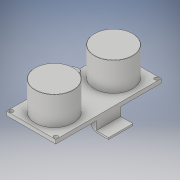
# Autodesk Inventor part: ultrasonicSensor
Saved by Autodesk Inventor 2018 (Build 220112000, 112)
## iProperties
Created: 2020-03-26
Part Number: ultrasonicSensor
Material: Generic
Document SubType Name: Modeling
Designer: natha
Density: 1 g/cm^3
Appearance: Default
Author: natha
Autodesk Inventor part; units mm, degrees
ref_plane "YZ Plane" through (0, 0, 0) normal (1, 0, 0) x (0, 1, 0)
ref_plane "XZ Plane" through (0, 0, 0) normal (0, 1, 0) x (-1, 0, 0)
ref_plane "XY Plane" through (0, 0, 0) normal (0, 0, 1) x (1, 0, 0)
sketch "Sketch1" plane through (0, 0, 0) normal (0, 1, 0) x (-1, 0, 0)
  line L0 (0, 0) -> (20.25, 0)
  line L1 (20.25, 0) -> (20.25, -43.35)
  line L2 (20.25, -43.35) -> (0, -43.35)
  line L3 (0, -43.35) -> (0, 0)
  dimension "d0" = 20.25
  dimension "d1" = 43.35
  constraints: 8 end point, 2 parallel, 1 horizontal, 1 perpendicular
  measures "d0" distance of L1.end L2.end
  measures "d1" distance of L0.end L1.end
extrude "Extrusion1" add sketch "Sketch1" along normal blind 1.6
sketch "Sketch2" plane through (0, 1.6, 0) normal (0, 1, 0) x (1, 0, 0)
  circle A0 centre (-19.25, 1) radius 0.8
  line L0 (-20.25, 43.35) -> (-20.25, 0) projected
  line L1 (-20.25, 0) -> (0, 0) projected
  circle A1 centre (-1, 1) radius 0.8
  line L2 (0, 0) -> (0, 43.35) projected
  circle A2 centre (-19.25, 42.35) radius 0.8
  line L3 (0, 43.35) -> (-20.25, 43.35) projected
  circle A3 centre (-1, 42.35) radius 0.8
  dimension "d4" = 1.6
  dimension "d5" = 1
  dimension "d6" = 1
  dimension "d7" = 1.6
  dimension "d8" = 1
  dimension "d9" = 1.6
  dimension "d10" = 1
  dimension "d11" = 1.6
  constraints: 4 centre point
  measures "d4" diameter of A0
  measures "d5" distance from line of L0 A0.centre
  measures "d6" distance from line of L1 A0.centre
  measures "d7" diameter of A1
  measures "d8" distance from line of A1.centre L2
  measures "d9" diameter of A2
  measures "d10" distance from line of L3 A2.centre
  measures "d11" diameter of A3
extrude "Extrusion2" cut sketch "Sketch2" against normal blind 1.6 contours A0 | A1 | A2 | A3
sketch "Sketch3" plane through (0, 1.6, 0) normal (0, 1, 0) x (1, 0, 0)
  line L0 (-19.75, 16.25) -> (-15.35, 16.25)
  line L1 (-15.35, 16.25) -> (-15.35, 27)
  line L2 (-15.35, 27) -> (-19.75, 27)
  line L3 (-19.75, 27) -> (-19.75, 16.25)
  line L4 (-20.25, 43.35) -> (-20.25, 0) projected
  line L5 (-20.25, 0) -> (0, 0) projected
  circle A0 centre (-10.125, 9.5) radius 7.875
  circle A1 centre (-10.125, 33.85) radius 7.875
  line L6 (0, 43.35) -> (-20.25, 43.35) projected
  dimension "d14" = 4.4
  dimension "d15" = 10.75
  dimension "d16" = 0.5
  dimension "d17" = 27
  dimension "d18" = 15.75
  dimension "d19" = 15.75
  dimension "d20" = 9.5
  dimension "d21" = 9.5
  dimension "d22" = 10.125
  dimension "d23" = 10.125
  constraints: 8 end point, 2 centre point, 2 parallel, 1 horizontal, 1 perpendicular
  measures "d14" distance of L2.end L1.end
  measures "d15" distance of L1.end L0.end
  measures "d16" distance between parallel lines of L4 L3
  measures "d17" distance between parallel lines of L5 L2
  measures "d18" diameter of A0
  measures "d19" diameter of A1
  measures "d20" distance from line of L5 A0.centre
  measures "d21" distance from line of L6 A1.centre
  measures "d22" distance from line of L4 A0.centre
  measures "d23" distance from line of L4 A1.centre
extrude "Extrusion3" add sketch "Sketch3" along normal blind 3.25
sketch "Sketch4" plane through (-10.125, 4.85, -9.5) normal (0, 1, 0) x (1, 0, 0)
  circle A0 centre (0, 0) radius 7.875
  point P0 (10.125, -9.5)
  constraints: 1 centre point
extrude "Extrusion4" add sketch "Sketch4" along normal blind 8.55
sketch "Sketch5" plane through (-10.125, 4.85, -33.85) normal (0, 1, 0) x (1, 0, 0)
  circle A0 centre (0, 0) radius 7.875
  point P0 (10.125, -33.85)
  constraints: 1 centre point
extrude "Extrusion5" add sketch "Sketch5" along normal blind 8.55
fillet "Fillet1" radius 2.2 4 edges at (-19.75, 3.225, -27) (-15.35, 3.225, -27) (-19.75, 3.225, -16.25) (-15.35, 3.225, -16.25)
fillet "Fillet2" radius 0.2 8 edges at (-19.1057, 4.85, -16.8943) (-17.55, 4.85, -16.25) (-15.9943, 4.85, -16.8943) (-15.35, 4.85, -21.625) (-19.1057, 4.85, -26.3557) (-17.55, 4.85, -27) (-15.9943, 4.85, -26.3557) (-19.75, 4.85, -21.625)
fillet "Fillet3" radius 0.1 2 edges at (-18, 13.4, -9.5) (-18, 13.4, -33.85)
sketch "Sketch6" plane through (0, 0, 0) normal (0, -1, 0) x (1, 0, 0)
  line L0 (0, -26.675) -> (-2.5, -26.675)
  line L1 (-2.5, -26.675) -> (-2.5, -16.675)
  line L2 (-2.5, -16.675) -> (0, -16.675)
  line L3 (0, -16.675) -> (0, -26.675)
  line L4 (-20.25, -43.35) -> (0, -43.35) projected
  point P0 (0, 0)
  dimension "d33" = 2.5
  dimension "d34" = 10
  dimension "d35" = 26.675
  constraints: 8 end point, 2 parallel, 1 horizontal, 1 perpendicular
  measures "d33" distance of L1.end L2.end
  measures "d34" distance of L0.end L1.end
  measures "d35" distance between parallel lines of L4 L2
extrude "Extrusion6" add sketch "Sketch6" along normal blind 4.25
sketch "Sketch7" plane through (0, 0, -43.35) normal (1, 0, 0) x (0, 0, -1)
  line L0 (-16.675, -4.25) -> (-26.675, -4.25) projected
  line L1 (-26.675, 0) -> (-26.675, -4.25) projected
  line L2 (-16.675, -4.25) -> (-26.675, -4.25)
  line L3 (-26.675, -4.25) -> (-26.675, -3.55)
  line L4 (-26.675, -3.55) -> (-16.675, -3.55)
  line L5 (-16.675, -3.55) -> (-16.675, -4.25)
  point P0 (-43.35, 0)
  dimension "d38" = 0.7
  constraints: 8 end point, 2 parallel, 1 horizontal, 1 perpendicular, 1 point on line
  measures "d38" distance of L2.end L3.end
extrude "Extrusion7" add sketch "Sketch7" along normal blind 5
fillet "Fillet4" radius 3 1 edges at (-2.5, -4.25, -21.675)
body "Solid1"
